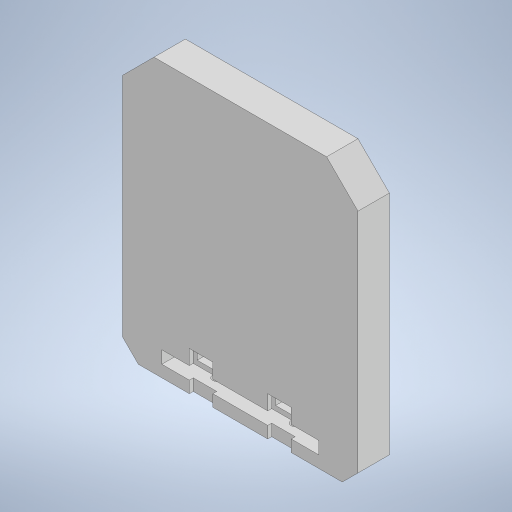
# Autodesk Inventor part: каретка_м2_без_м
Saved by Autodesk Inventor 2023.1 (Build 271208000, 208)
## iProperties
Created: 2025-12-14
Part Number: каретка_м2_без_м
Material: Типовые
Document SubType Name: Modeling
Designer: DELL
Density: 1 g/cm^3
Appearance: По умолчанию
Author: DELL
Autodesk Inventor part; units mm, degrees
ref_plane "YZ Plane" through (0, 0, 0) normal (1, 0, 0) x (0, 1, 0)
ref_plane "XZ Plane" through (0, 0, 0) normal (0, 1, 0) x (-1, 0, 0)
ref_plane "XY Plane" through (0, 0, 0) normal (0, 0, 1) x (1, 0, 0)
sketch "Эскиз1" plane through (0, 0, 0) normal (0, 0, 1) x (1, 0, 0)
  line L0 (16.9838, 20.6364) -> (20.6364, 16.9838) projected
  arc A0 (16.9838, 20.6364) -> (16.3474, 20.9) centre (16.3474, 20) ccw projected
  line L1 (-16.3474, 20.9) -> (16.3474, 20.9) projected
  arc A1 (-16.3474, 20.9) -> (-16.9838, 20.6364) centre (-16.3474, 20) ccw projected
  line L2 (-20.6364, 16.9838) -> (-16.9838, 20.6364) projected
  arc A2 (-20.6364, 16.9838) -> (-20.9, 16.3474) centre (-20, 16.3474) ccw projected
  line L3 (-20.9, -16.3474) -> (-20.9, 16.3474) projected
  arc A3 (-20.9, -16.3474) -> (-20.6364, -16.9838) centre (-20, -16.3474) ccw projected
  line L4 (-16.9838, -20.6364) -> (-20.6364, -16.9838) projected
  arc A4 (-16.9838, -20.6364) -> (-16.3474, -20.9) centre (-16.3474, -20) ccw projected
  line L5 (16.3474, -20.9) -> (-16.3474, -20.9) projected
  arc A5 (16.3474, -20.9) -> (16.9838, -20.6364) centre (16.3474, -20) ccw projected
  line L6 (20.6364, -16.9838) -> (16.9838, -20.6364) projected
  arc A6 (20.6364, -16.9838) -> (20.9, -16.3474) centre (20, -16.3474) ccw projected
  line L7 (20.9, 16.3474) -> (20.9, -16.3474) projected
  arc A7 (20.9, 16.3474) -> (20.6364, 16.9838) centre (20, 16.3474) ccw projected
  circle A8 centre (15.5574, -15.5574) radius 1.45 projected
  circle A9 centre (0, 0) radius 11 projected
  circle A10 centre (-15.5574, -15.5574) radius 1.45 projected
  circle A11 centre (-15.5574, 15.5574) radius 1.45 projected
  circle A12 centre (15.5574, 15.5574) radius 1.45 projected
  point P0 (0, 0)
extrude "Выдавливание1" add sketch "Эскиз1" along normal blind 3
sketch "Эскиз2" plane through (0, 0, 3) normal (0, 0, 1) x (1, 0, 0)
  line L0 (16.3474, 20.9) -> (-16.3474, 20.9) construction
  line L1 (-30, -20.9) -> (30, -20.9)
  line L2 (30, -20.9) -> (30, 20.9)
  line L3 (30, 20.9) -> (-30, 20.9)
  line L4 (-30, 20.9) -> (-30, -20.9)
  circle A0 centre (0, 0) radius 11 construction
  line L5 (-30, -20.9) -> (30, 20.9) construction
  line L6 (30, -20.9) -> (-30, 20.9) construction
  line L7 (-30, -20.9) -> (30, -20.9)
  line L8 (30, -20.9) -> (30, -48.9)
  line L9 (30, -48.9) -> (-30, -48.9)
  line L10 (-30, -48.9) -> (-30, -20.9)
  line L11 (-16.9838, 20.6364) -> (-20.6364, 16.9838) projected
  arc A1 (-20.6364, 16.9838) -> (-20.9, 16.3474) centre (-20, 16.3474) ccw projected
  line L12 (-20.9, 16.3474) -> (-20.9, -16.3474) projected
  arc A2 (-20.9, -16.3474) -> (-20.6364, -16.9838) centre (-20, -16.3474) ccw projected
  line L13 (-20.6364, -16.9838) -> (-16.9838, -20.6364) projected
  arc A3 (-16.9838, -20.6364) -> (-16.3474, -20.9) centre (-16.3474, -20) ccw projected
  line L14 (-16.3474, -20.9) -> (16.3474, -20.9) projected
  arc A4 (16.3474, -20.9) -> (16.9838, -20.6364) centre (16.3474, -20) ccw projected
  line L15 (16.9838, -20.6364) -> (20.6364, -16.9838) projected
  arc A5 (20.6364, -16.9838) -> (20.9, -16.3474) centre (20, -16.3474) ccw projected
  line L16 (20.9, -16.3474) -> (20.9, 16.3474) projected
  arc A6 (20.9, 16.3474) -> (20.6364, 16.9838) centre (20, 16.3474) ccw projected
  line L17 (20.6364, 16.9838) -> (16.9838, 20.6364) projected
  arc A7 (16.9838, 20.6364) -> (16.3474, 20.9) centre (16.3474, 20) ccw projected
  line L18 (16.3474, 20.9) -> (-16.3474, 20.9) projected
  arc A8 (-16.3474, 20.9) -> (-16.9838, 20.6364) centre (-16.3474, 20) ccw projected
  circle A9 centre (0, 0) radius 11 construction
  circle A10 centre (15.5574, 15.5574) radius 1.45 construction
  circle A11 centre (-15.5574, 15.5574) radius 1.45 construction
  circle A12 centre (-15.5574, -15.5574) radius 1.45 construction
  circle A13 centre (15.5574, -15.5574) radius 1.45 construction
  dimension "d4" = 60
  dimension "d5" = 60
  dimension "d6" = 28
  constraints: 20 end point, 4 parallel, 2 horizontal, 2 midpoint, 2 perpendicular
  measures "d4" distance of L3.end L2.end
  measures "d5" distance of L8.end L9.end
  measures "d6" distance of L7.end L8.end
extrude "Выдавливание2" add sketch "Эскиз2" against normal blind 8
ref_plane "РабПлоскость4" through (-23, -29.9, -1) normal (0, -1, 0) x (1, 0, 0)
chamfer "Фаска1" distance 4 angle 45 2 edges at (30, -48.9, -1) (-30, -48.9, -1)
chamfer "Фаска2" distance 8 angle 45 2 edges at (30, 20.9, -1) (-30, 20.9, -1)
sketch "Эскиз14" plane through (-30, -44.9, -5) normal (-1, 0, 0) x (0, 0, 1)
  line L0 (0, 57.8) -> (8, 57.8) construction
  line L1 (0, 0) -> (0, 57.8) construction
  line L2 (8, 0) -> (0, 0) construction
  line L3 (8, 57.8) -> (8, 0) construction
  line L4 (8, 57.8) -> (0, 57.8) projected
  line L5 (4, 57.8) -> (4, 0) construction
  line L6 (8, 0) -> (0, 0) projected
  circle A0 centre (4, 47.8) radius 2
  circle A1 centre (4, 33.8) radius 2
  dimension "d107" = 4
  dimension "d108" = 4
  dimension "d109" = 10
  dimension "d113" = 14
  constraints: 2 centre point, 2 end point, 2 midpoint, 2 point on line
  measures "d107" diameter of A0
  measures "d108" diameter of A1
  measures "d109" distance from line of L0 A0.centre
  measures "d113" distance of A1.centre A0.centre
extrude "Выдавливание13" cut sketch "Эскиз14" against normal blind 6
sketch "Эскиз25" plane through (0, 0, 3) normal (0, 0, 1) x (1, 0, 0)
  line L0 (-20, -42.7) -> (20, -42.7)
  line L1 (20, -42.7) -> (20, -45.9)
  line L2 (20, -45.9) -> (-20, -45.9)
  line L3 (-20, -45.9) -> (-20, -42.7)
  line L4 (-20, -42.7) -> (20, -45.9) construction
  line L5 (20, -42.7) -> (-20, -45.9) construction
  line L6 (-26, -48.9) -> (26, -48.9) construction
  line L7 (26, -48.9) -> (-26, -48.9) projected
  line L8 (0, -48.9) -> (0, 20.9) construction
  line L9 (16.3474, 20.9) -> (-16.3474, 20.9) construction
  point P0 (0, 0)
  point P1 (0, -44.3)
  dimension "d170" = 40
  dimension "d171" = 3.2
  dimension "d172" = 3
  constraints: 14 end point, 4 midpoint, 2 parallel, 1 horizontal, 1 perpendicular, 1 point on line
  measures "d170" distance of L1.end L2.end
  measures "d171" distance of L0.end L1.end
  measures "d172" distance between parallel lines of L6 L2
extrude "Выдавливание25" cut sketch "Эскиз25" against normal blind 8
sketch "Эскиз27" plane through (-26, -48.9, 3) normal (0, -1, 0) x (1, 0, 0)
  line L0 (0, -8) -> (0, 0) construction
  line L1 (52, 0) -> (52, -8) construction
  line L2 (0, -4) -> (52, -4) construction
  circle A0 centre (16, -4) radius 1.1
  line L3 (46, 0) -> (46, -8) construction
  line L4 (6, 0) -> (46, 0) construction
  line L5 (46, 0) -> (46, -8) construction
  line L6 (46, -8) -> (6, -8) construction
  line L7 (6, -8) -> (6, 0) construction
  line L8 (6, 0) -> (46, -8) construction
  line L9 (46, 0) -> (6, -8) construction
  circle A1 centre (36, -4) radius 1.1
  point P0 (26, -4)
  dimension "d177" = 2.2
  dimension "d178" = 10
  dimension "d179" = 2.2
  dimension "d180" = 10
  constraints: 14 end point, 5 midpoint, 2 centre point, 2 parallel, 2 point on line, 1 horizontal, 1 perpendicular
  measures "d177" diameter of A0
  measures "d178" distance from line of L7 A0.centre
  measures "d179" diameter of A1
  measures "d180" distance from line of L3 A1.centre
extrude "Выдавливание26" cut sketch "Эскиз27" against normal blind 14
sketch "Эскиз28" plane through (0, 0, 3) normal (0, 0, 1) x (1, 0, 0)
  line L0 (20, -45.9) -> (-20, -45.9) construction
  line L1 (-20, -45.9) -> (-20, -42.7) construction
  line L2 (-20, -42.7) -> (20, -42.7) construction
  line L3 (20, -42.7) -> (20, -45.9) construction
  line L4 (-26, -48.9) -> (26, -48.9) projected
  line L5 (-13, -48.9) -> (-7, -48.9)
  line L6 (-7, -48.9) -> (-7, -38.9)
  line L7 (-7, -38.9) -> (-13, -38.9)
  line L8 (-13, -38.9) -> (-13, -48.9)
  line L9 (-10, -38.9) -> (-10, -48.9) construction
  point P0 (0, 0)
  point P1 (-10, -43.9)
  point P2 (-20, -44.3)
  dimension "d183" = 6
  dimension "d184" = 10
  dimension "d185" = 10
  constraints: 10 end point, 4 midpoint, 2 parallel, 1 horizontal, 1 perpendicular, 1 point on line
  measures "d183" distance of L7.end L6.end
  measures "d184" distance of L6.end L5.end
  measures "d185" horizontal distance of point (-10, -43.9) point (-20, -44.3)
extrude "Выдавливание27" cut sketch "Эскиз28" against normal blind 1
ref_plane "РабПлоскость8" through (0, 0, -1) normal (0, 0, -1) x (-1, 0, 0)
mirror "Зеркальное отражение4" about plane through (0, 0, 0) normal (1, 0, 0) of "Выдавливание27"
mirror "Зеркальное отражение5" about plane through (0, 0, -1) normal (0, 0, -1) of "Выдавливание27", "Зеркальное отражение4"
sketch "Эскиз29" plane through (0, 0, 2) normal (0, 0, 1) x (1, 0, 0)
  line L0 (-13, -38.9) -> (-7, -38.9) construction
  line L1 (-13, -42.7) -> (-13, -38.9) construction
  line L2 (7, -42.7) -> (7, -38.9) construction
  line L3 (7, -38.9) -> (13, -38.9) construction
  line L4 (-13, -38.9) -> (-7, -38.9) projected
  line L5 (-10, -38.9) -> (-10, -42.7) construction
  line L6 (-12, -39.9) -> (-8, -39.9)
  line L7 (-8, -39.9) -> (-8, -41.5)
  line L8 (-8, -41.5) -> (-12, -41.5)
  line L9 (-12, -41.5) -> (-12, -39.9)
  line L10 (-12, -39.9) -> (-8, -41.5) construction
  line L11 (-8, -39.9) -> (-12, -41.5) construction
  line L12 (-13, -42.7) -> (-7, -42.7) projected
  line L13 (7, -48.9) -> (-7, -48.9) construction
  line L14 (0, -48.9) -> (0, -38.1038) construction
  line L15 (12, -39.9) -> (8, -39.9)
  line L16 (8, -39.9) -> (8, -41.5)
  line L17 (8, -41.5) -> (12, -41.5)
  line L18 (12, -41.5) -> (12, -39.9)
  point P0 (0, 0)
  point P1 (-10, -40.7)
  dimension "d188" = 4
  dimension "d189" = 1.6
  dimension "d190" = 1.2
  constraints: 24 end point, 4 midpoint, 4 symmetric about line, 2 parallel, 2 vertical, 1 horizontal, 1 perpendicular, 1 point on line
  measures "d188" distance of L7.end L8.end
  measures "d189" distance of L6.end L7.end
  measures "d190" distance between parallel lines of L12 L8
extrude "Выдавливание28" cut sketch "Эскиз29" against normal blind 10
